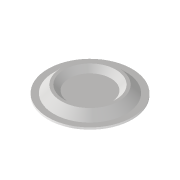
# Autodesk Inventor part: 50_ETL_Membrane_v0
Saved by Autodesk Inventor 2022 (Build 260153000, 153)
## iProperties
Created: 2021-12-31
Part Number: 50_ETL_Membrane_v0
Material: Generisch
Document SubType Name: Modeling
Designer: diederichbenedict
Density: 1 g/cm^3
Appearance: Vorgabe
Author: diederichbenedict
Autodesk Inventor part; units mm, degrees
ref_plane "YZ Plane" through (0, 0, 0) normal (1, 0, 0) x (0, 1, 0)
ref_plane "XZ Plane" through (0, 0, 0) normal (0, 1, 0) x (-1, 0, 0)
ref_plane "XY Plane" through (0, 0, 0) normal (0, 0, 1) x (1, 0, 0)
sketch "Skizze1" plane through (0, 0, 0) normal (1, 0, 0) x (0, 1, 0)
  line L0 (3, 8.0893) -> (5.1212, 8.0893) construction
  line L1 (-0.0509, -6) -> (0.0741, -6) construction
  line L2 (0.0741, -6) -> (0.0741, 6) construction
  line L3 (0.0741, 6) -> (-0.0509, 6) construction
  line L4 (-0.0509, 6) -> (-0.0509, -6) construction
  line L5 (-0.0509, -6) -> (0.0741, 6) construction
  line L6 (0.0741, -6) -> (-0.0509, 6) construction
  line L7 (-0.0509, 6) -> (-0.0509, 0)
  line L8 (-0.0509, 0) -> (-0.3509, 0)
  line L9 (-0.3509, 0) -> (-0.3509, 6.7569)
  line L10 (-0.3509, 6.7569) -> (0.8491, 7.9569)
  line L11 (0.8491, 7.9569) -> (0.8491, 8.3023)
  line L12 (-0.0509, 6) -> (-0.0509, 6.2)
  line L13 (-0.0509, 6.2) -> (1.4491, 7.7)
  line L14 (1.4491, 7.7) -> (1.4491, 8.5508)
  line L15 (1.4491, 8.5508) -> (-0.7509, 10.7508)
  line L16 (-1.3509, 12.5) -> (-1.3509, 9.3023)
  line L17 (0.8491, 8.3023) -> (-0.1509, 9.3023)
  line L18 (-0.1509, 9.3023) -> (-1.3509, 9.3023)
  line L19 (-0.7509, 10.7508) -> (-0.7509, 12.5)
  line L20 (-0.7509, 12.5) -> (-1.3509, 12.5)
  point P0 (0.0116, 0)
  point P1 (0.0116, 0)
  dimension "d14" = 0.125
  dimension "d15" = 12
  dimension "d16" = 0.3
  dimension "d18" = 135
  dimension "d20" = 0.2
  dimension "d27" = 135
  dimension "d28" = 1
  dimension "d29" = 1.2
  dimension "d30" = 0.6
  dimension "d31" = 0.6
  dimension "d34" = 1
  dimension "d36" = 0.6
  dimension "d37" = 12.5
  constraints: 42 end point, 5 midpoint, 4 horizontal, 4 parallel, 4 perpendicular, 3 vertical
  measures "d14" distance of L3.end L2.end
  measures "d15" distance of L2.end L1.end
  measures "d16" distance of L7.end L8.end
  measures "d18" angle of L9 L10
  measures "d20" distance of L3.end L12.end
  measures "d27" angle of L11 L17
  measures "d28" distance from line of L17.end L11
  measures "d29" distance between parallel lines of L9 L11
  measures "d30" distance between parallel lines of L11 L14
  measures "d31" distance between parallel lines of L15 L17
  measures "d34" distance between parallel lines of L9 L16
  measures "d36" distance between parallel lines of L19 L16
  measures "d37" distance between parallel lines of L8 L20
revolve "Umdrehung1" add sketch "Skizze1" angle 360 about axis through (0, -0.0509, 0) along (0, -1, 0)
